Autodesk Fusion 360 part; units mm, degrees
(part 5 of 9)
  line L160 (103.5375, 54.625) -> (115.5375, 54.625)
  arc A163 (116.5375, 53.625) -> (115.5375, 54.625) centre (115.5375, 53.625) ccw
  line L161 (116.5375, 53.625) -> (116.5375, 41.625)
  arc A164 (115.5375, 40.625) -> (116.5375, 41.625) centre (115.5375, 41.625) ccw
  line L162 (115.5375, 40.625) -> (103.5375, 40.625)
  arc A165 (102.5375, 41.625) -> (103.5375, 40.625) centre (103.5375, 41.625) ccw
  line L163 (102.5375, 41.625) -> (102.5375, 53.625)
  arc A166 (251.175, 16.525) -> (250.175, 15.525) centre (251.175, 15.525) ccw
  line L164 (251.175, 16.525) -> (263.175, 16.525)
  arc A167 (264.175, 15.525) -> (263.175, 16.525) centre (263.175, 15.525) ccw
  line L165 (264.175, 15.525) -> (264.175, 3.525)
  arc A168 (263.175, 2.525) -> (264.175, 3.525) centre (263.175, 3.525) ccw
  line L166 (263.175, 2.525) -> (251.175, 2.525)
  arc A169 (250.175, 3.525) -> (251.175, 2.525) centre (251.175, 3.525) ccw
  line L167 (250.175, 3.525) -> (250.175, 15.525)
  arc A170 (123.2563, 72.675) -> (122.2563, 73.675) centre (122.2563, 72.675) ccw
  line L168 (123.2563, 72.675) -> (123.2563, 60.675)
  arc A171 (122.2563, 59.675) -> (123.2563, 60.675) centre (122.2563, 60.675) ccw
  line L169 (122.2563, 59.675) -> (92.0563, 59.675)
  arc A172 (91.0563, 60.675) -> (92.0563, 59.675) centre (92.0563, 60.675) ccw
  line L170 (91.0563, 60.675) -> (91.0563, 72.675)
  arc A173 (92.0563, 73.675) -> (91.0563, 72.675) centre (92.0563, 72.675) ccw
  line L171 (92.0563, 73.675) -> (122.2563, 73.675)
  circle A174 centre (128.588, 37.025) radius 1.25
  circle A175 centre (47.625, 9.525) radius 1.25
  arc A176 (132.1125, 35.575) -> (131.1125, 34.575) centre (132.1125, 34.575) ccw
  line L172 (132.1125, 35.575) -> (144.1125, 35.575)
  arc A177 (145.1125, 34.575) -> (144.1125, 35.575) centre (144.1125, 34.575) ccw
  line L173 (145.1125, 34.575) -> (145.1125, 22.575)
  arc A178 (144.1125, 21.575) -> (145.1125, 22.575) centre (144.1125, 22.575) ccw
  line L174 (144.1125, 21.575) -> (132.1125, 21.575)
  arc A179 (131.1125, 22.575) -> (132.1125, 21.575) centre (132.1125, 22.575) ccw
  line L175 (131.1125, 22.575) -> (131.1125, 34.575)
  arc A180 (94.0125, 35.575) -> (93.0125, 34.575) centre (94.0125, 34.575) ccw
  line L176 (94.0125, 35.575) -> (106.0125, 35.575)
  arc A181 (107.0125, 34.575) -> (106.0125, 35.575) centre (106.0125, 34.575) ccw
  line L177 (107.0125, 34.575) -> (107.0125, 22.575)
  arc A182 (106.0125, 21.575) -> (107.0125, 22.575) centre (106.0125, 22.575) ccw
  line L178 (106.0125, 21.575) -> (94.0125, 21.575)
  arc A183 (93.0125, 22.575) -> (94.0125, 21.575) centre (94.0125, 22.575) ccw
  line L179 (93.0125, 22.575) -> (93.0125, 34.575)
  circle A184 centre (32.525, 66.675) radius 1.25
  line L180 (241.3625, 58.15) -> (241.3625, 73.2)
  arc A185 (241.3625, 73.2) -> (239.8875, 74.675) centre (239.8875, 73.2) ccw
  line L181 (239.8875, 74.675) -> (12.525, 74.675)
  arc A186 (12.525, 74.675) -> (11.05, 73.2) centre (12.525, 73.2) ccw
  line L182 (11.05, 73.2) -> (11.05, 58.15)
  arc A187 (8.525, 55.625) -> (11.05, 58.15) centre (8.525, 58.15) ccw
  line L183 (8.525, 55.625) -> (3, 55.625)
  arc A188 (3, 55.625) -> (1.525, 54.15) centre (3, 54.15) ccw
  line L184 (1.525, 54.15) -> (1.525, 3)
  arc A189 (1.525, 3) -> (3, 1.525) centre (3, 3) ccw
  line L185 (3, 1.525) -> (263.7, 1.525)
  arc A190 (263.7, 1.525) -> (265.175, 3) centre (263.7, 3) ccw
  line L186 (265.175, 3) -> (265.175, 54.15)
  arc A191 (265.175, 54.15) -> (263.7, 55.625) centre (263.7, 54.15) ccw
  line L187 (263.7, 55.625) -> (243.8875, 55.625)
  arc A192 (241.3625, 58.15) -> (243.8875, 55.625) centre (243.8875, 58.15) ccw
  line L188 (163.7375, 72.3724) -> (155.7375, 72.3724)
  line L189 (155.7375, 72.3724) -> (155.7375, 74.675)
  line L190 (156.7375, 75.675) -> (162.7375, 75.675)
  line L191 (163.7375, 74.675) -> (163.7375, 72.3724)
  arc A193 (163.7375, 74.675) -> (162.7375, 75.675) centre (162.7375, 74.675) ccw
  arc A194 (156.7375, 75.675) -> (155.7375, 74.675) centre (156.7375, 74.675) ccw
  line L192 (131.5375, 70.0356) -> (139.5375, 70.0356)
  line L193 (139.5375, 70.0356) -> (139.5375, 74.675)
  line L194 (138.5375, 75.675) -> (132.5375, 75.675)
  line L195 (131.5375, 74.675) -> (131.5375, 70.0356)
  arc A195 (139.5375, 74.675) -> (138.5375, 75.675) centre (138.5375, 74.675) ccw
  arc A196 (132.5375, 75.675) -> (131.5375, 74.675) centre (132.5375, 74.675) ccw
  line L196 (150.1375, 73.675) -> (145.1375, 73.675)
  line L197 (145.1375, 73.675) -> (145.1375, 74.675)
  line L198 (145.1375, 74.675) -> (150.1375, 74.675)
  line L199 (150.1375, 74.675) -> (150.1375, 73.675)
  line L200 (90.0563, 55.625) -> (90.0563, 58.675)
  line L201 (164.7375, 58.675) -> (164.7375, 55.625)
  line L202 (134.1008, 59.675) -> (120, 59.675)
  line L203 (120, 59.675) -> (120, 62.425)
  line L204 (120, 62.425) -> (134.1008, 62.425)
  line L205 (134.1008, 62.425) -> (134.1008, 59.675)
  line L206 (91.0563, 69.6315) -> (99.0563, 69.6315)
  line L207 (99.0563, 69.6315) -> (99.0563, 74.675)
  line L208 (98.0563, 75.675) -> (92.0563, 75.675)
  line L209 (91.0563, 74.675) -> (91.0563, 69.6315)
  line L210 (123.2563, 68.7427) -> (115.2563, 68.7427)
  line L211 (115.2563, 68.7427) -> (115.2563, 74.675)
  line L212 (116.2563, 75.675) -> (122.2563, 75.675)
  line L213 (123.2563, 74.675) -> (123.2563, 68.7427)
  line L214 (109.6563, 73.675) -> (104.6563, 73.675)
  line L215 (104.6563, 73.675) -> (104.6563, 74.675)
  line L216 (104.6563, 74.675) -> (109.6563, 74.675)
  line L217 (109.6563, 74.675) -> (109.6563, 73.675)
  line L218 (91.0563, 61.8134) -> (91.0563, 59.675)
  line L219 (91.0563, 59.675) -> (91.0563, 59.675)
  arc A197 (91.0563, 59.675) -> (90.0563, 58.675) centre (91.0563, 58.675) ccw
  line L220 (92.0563, 59.675) -> (122.2563, 59.675)
  line L221 (163.7375, 61.2223) -> (163.7375, 59.675)
  line L222 (132.5375, 59.675) -> (162.7375, 59.675)
  line L223 (163.7375, 59.675) -> (163.7375, 59.675)
  arc A198 (164.7375, 58.675) -> (163.7375, 59.675) centre (163.7375, 58.675) ccw
  line L224 (159.6875, 52.1672) -> (154.6375, 52.1672)
  line L225 (154.6375, 52.1672) -> (154.6375, 53.625)
  line L226 (155.6375, 54.625) -> (158.6875, 54.625)
  line L227 (159.6875, 53.625) -> (159.6875, 52.1672)
  arc A199 (159.6875, 53.625) -> (158.6875, 54.625) centre (158.6875, 53.625) ccw
  arc A200 (155.6375, 54.625) -> (154.6375, 53.625) centre (155.6375, 53.625) ccw
  line L228 (164.7375, 54.625) -> (160.6875, 54.625)
  line L229 (158.6875, 54.625) -> (155.6375, 54.625)
  line L230 (140.6375, 52.2028) -> (135.5875, 52.2028)
  line L231 (135.5875, 52.2028) -> (135.5875, 53.625)
  line L232 (136.5875, 54.625) -> (139.6375, 54.625)
  line L233 (140.6375, 53.625) -> (140.6375, 52.2028)
  arc A201 (140.6375, 53.625) -> (139.6375, 54.625) centre (139.6375, 53.625) ccw
  arc A202 (136.5875, 54.625) -> (135.5875, 53.625) centre (136.5875, 53.625) ccw
  line L234 (153.6375, 54.625) -> (141.6375, 54.625)
  line L235 (139.6375, 54.625) -> (136.5875, 54.625)
  line L236 (121.5875, 52.4995) -> (116.5375, 52.4995)
  line L237 (116.5375, 52.4995) -> (116.5375, 53.625)
  line L238 (117.5375, 54.625) -> (120.5875, 54.625)
  line L239 (121.5875, 53.625) -> (121.5875, 52.4995)
  arc A203 (121.5875, 53.625) -> (120.5875, 54.625) centre (120.5875, 53.625) ccw
  arc A204 (117.5375, 54.625) -> (116.5375, 53.625) centre (117.5375, 53.625) ccw
  line L240 (134.5875, 54.625) -> (122.5875, 54.625)
  line L241 (120.5875, 54.625) -> (117.5375, 54.625)
  line L242 (102.5375, 52.5305) -> (97.4875, 52.5305)
  line L243 (97.4875, 52.5305) -> (97.4875, 53.625)
  line L244 (98.4875, 54.625) -> (101.5375, 54.625)
  line L245 (102.5375, 53.625) -> (102.5375, 52.5305)
  arc A205 (102.5375, 53.625) -> (101.5375, 54.625) centre (101.5375, 53.625) ccw
  arc A206 (98.4875, 54.625) -> (97.4875, 53.625) centre (98.4875, 53.625) ccw
  line L246 (96.4875, 54.625) -> (90.0563, 54.625)
  line L247 (115.5375, 54.625) -> (103.5375, 54.625)
  line L248 (101.5375, 54.625) -> (98.4875, 54.625)
  arc A207 (123.2563, 74.675) -> (122.2563, 75.675) centre (122.2563, 74.675) ccw
  arc A208 (116.2563, 75.675) -> (115.2563, 74.675) centre (116.2563, 74.675) ccw
  arc A209 (99.0563, 74.675) -> (98.0563, 75.675) centre (98.0563, 74.675) ccw
  arc A210 (92.0563, 75.675) -> (91.0563, 74.675) centre (92.0563, 74.675) ccw
  line L249 (169.1875, 54.625) -> (164.1875, 54.625)
  line L250 (164.7375, 55.625) -> (169.1875, 55.625)
  line L251 (169.1875, 55.625) -> (169.1875, 54.625)
  line L252 (87.9875, 54.625) -> (92.9875, 54.625)
  line L253 (90.0563, 55.625) -> (87.9875, 55.625)
  line L254 (87.9875, 55.625) -> (87.9875, 54.625)
  dimension "d114" = 8
  dimension "d115" = 2
  dimension "d116" = 1
  dimension "d117" = 8
  dimension "d118" = 2
  dimension "d119" = 1
  dimension "d120" = 5
  dimension "d121" = 13.6
  dimension "d122" = 1
  dimension "d123" = 1
  dimension "d124" = 2.75
  dimension "d125" = 8
  dimension "d126" = 2
  dimension "d127" = 8
  dimension "d128" = 2
  dimension "d129" = 5
  dimension "d130" = 13.6
  dimension "d131" = 1
  dimension "d132" = 1
  dimension "d133" = 1
  dimension "d134" = 1
  dimension "d135" = 1
  dimension "d136" = 1
  dimension "d137" = 1
  dimension "d138" = 5
  dimension "d139" = 1
  dimension "d140" = 4.5
  dimension "d141" = 5
  dimension "d142" = 1
  dimension "d143" = 4.5
  constraint horizontal L188
  constraint vertical L189
  constraint horizontal L190
  constraint vertical L191
  constraint coincident L130 L188.start
  constraint tangent L190 A193
  constraint tangent L191 A193
  constraint tangent L189 A194
  constraint tangent L190 A194
  constraint equal A193 A194
  constraint horizontal L192
  constraint vertical L193
  constraint horizontal L194
  constraint vertical L195
  constraint coincident L128 L192.start
  constraint tangent L193 A195
  constraint tangent L194 A195
  constraint tangent L194 A196
  constraint tangent L195 A196
  constraint equal A195 A196
  constraint horizontal L196
  constraint vertical L197
  constraint horizontal L198
  constraint vertical L199
  constraint coincident L129 L196.start
  constraint horizontal L228
  constraint vertical L200
  constraint vertical L201
  constraint coincident L156 L228.start
  constraint horizontal L202
  constraint vertical L203
  constraint horizontal L204
  constraint vertical L205
  constraint coincident L131 L202.start
  constraint horizontal L206
  constraint vertical L207
  constraint horizontal L208
  constraint vertical L209
  constraint coincident L170 L206.start
  constraint horizontal L210
  constraint vertical L211
  constraint horizontal L212
  constraint vertical L213
  constraint coincident L168 L210.start
  constraint horizontal L214
  constraint vertical L215
  constraint horizontal L216
  constraint vertical L217
  constraint coincident L171 L214.start
  constraint coincident L170 L218.start
  constraint parallel L170 L218
  constraint tangent L200 A197
  constraint collinear L220 L222
  constraint coincident L130 L221.start
  constraint parallel L130 L221
  constraint coincident L221.end L222
  constraint tangent L201 A198
  constraint horizontal L224
  constraint vertical L225
  constraint horizontal L226
  constraint vertical L227
  constraint coincident L159 L224.start
  constraint tangent L226 A199
  constraint tangent L227 A199
  constraint tangent L225 A200
  constraint tangent L226 A200
  constraint equal A199 A200
  constraint collinear L228 L229
  constraint collinear L229 L234
  constraint horizontal L230
  constraint vertical L231
  constraint horizontal L232
  constraint vertical L233
  constraint coincident L139 L230.start
  constraint tangent L232 A201
  constraint tangent L233 A201
  constraint tangent L231 A202
  constraint tangent L232 A202
  constraint equal A201 A202
  constraint collinear L234 L235
  constraint collinear L235 L240
  constraint horizontal L236
  constraint vertical L237
  constraint horizontal L238
  constraint vertical L239
  constraint coincident L155 L236.start
  constraint tangent L238 A203
  constraint tangent L239 A203
  constraint tangent L237 A204
  constraint tangent L238 A204
  constraint equal A203 A204
  constraint collinear L240 L241
  constraint collinear L241 L247
  constraint horizontal L242
  constraint vertical L243
  constraint horizontal L244
  constraint vertical L245
  constraint coincident L163 L242.start
  constraint tangent L244 A205
  constraint tangent L245 A205
  constraint tangent L243 A206
  constraint tangent L244 A206
  constraint equal A205 A206
  constraint collinear L246 L247
  constraint collinear L247 L248
  constraint tangent L212 A207
  constraint tangent L213 A207
  constraint tangent L211 A208
  constraint tangent L212 A208
  constraint equal A207 A208
  constraint tangent L207 A209
  constraint tangent L208 A209
  constraint equal A207 A209
  constraint tangent L208 A210
  constraint tangent L209 A210
  constraint equal A207 A210
  constraint horizontal L249
  constraint horizontal L250
  constraint vertical L251
  constraint coincident L156 L249.start
  constraint horizontal L252
  constraint horizontal L253
  constraint vertical L254
  constraint coincident L112 L252.start
  measures "d114" distance of L188.start L188.end
  measures "d115" distance of L129 L190
  measures "d116" radius of A193
  measures "d117" distance of L192.start L192.end
  measures "d118" distance of L129 L194
  measures "d119" radius of A195
  measures "d120" distance of L196.start L196.end
  measures "d121" distance of L130 L199
  measures "d122" distance of L170 L200
  measures "d123" distance of L130 L201
  measures "d124" distance of L202.start L204.end
  measures "d125" distance of L206.start L206.end
  measures "d126" distance of L171 L208
  measures "d127" distance of L210.start L210.end
  measures "d128" distance of L171 L212
  measures "d129" distance of L214.start L214.end
  measures "d130" distance of L168 L217
  measures "d131" radius of A197
  measures "d132" radius of A198
  measures "d133" radius of A199
  measures "d134" radius of A201
  measures "d135" radius of A203
  measures "d136" radius of A205
  measures "d137" radius of A207
  measures "d138" distance of L249.start L249.end
  measures "d139" distance of L249.start L250.end
  measures "d140" distance of L157 L251
  measures "d141" distance of L252.start L252.end
  measures "d142" distance of L252.start L253.end
  measures "d143" distance of L115 L254
extrude "Extrude7" cut sketch "Sketch8" against normal blind 3 contours L112 A113 A133 L131 A138 L136 A139 A154 L152 A155 A158 L156 A162 L160 A163 L169 A172 L200 L201 L202 L218 A197 L220 L221 L222 A198 L226 A199 A200 L228 L229 L232 A201 A202 L234 L235 L238 A203 A204 L240 L241 L244 A205 A206 L246 L247 L248 L249 L250 L251 L252 L253 L254 | A130 L128 L168 A171 L202 L204 | A173 L171 L181 L207 L209 | L171 L181 L214 L215 L216 L217 | A170 L171 L181 L211 L213 | A131 L129 L181 L193 L195 | L129 L181 L196 L197 L198 L199 | L129 A132 L181 L189 L191
sketch "Sketch9" plane through (0, 0, 0) normal (0, -1, 0) x (1, 0, 0)
  arc A0 (241.3625, 73.2) -> (239.8875, 74.675) centre (239.8875, 73.2) ccw
  line L0 (241.3625, 73.2) -> (241.3625, 58.15)
  arc A1 (241.3625, 58.15) -> (243.8875, 55.625) centre (243.8875, 58.15) ccw
  line L1 (243.8875, 55.625) -> (263.7, 55.625)
  arc A2 (265.175, 54.15) -> (263.7, 55.625) centre (263.7, 54.15) ccw
  line L2 (265.175, 54.15) -> (265.175, 3)
  arc A3 (263.7, 1.525) -> (265.175, 3) centre (263.7, 3) ccw
  line L3 (263.7, 1.525) -> (3, 1.525)
  arc A4 (1.525, 3) -> (3, 1.525) centre (3, 3) ccw
  line L4 (1.525, 3) -> (1.525, 54.15)
  arc A5 (3, 55.625) -> (1.525, 54.15) centre (3, 54.15) ccw
  line L5 (3, 55.625) -> (8.525, 55.625)
  arc A6 (8.525, 55.625) -> (11.05, 58.15) centre (8.525, 58.15) ccw
  line L6 (11.05, 58.15) -> (11.05, 73.2)
  arc A7 (12.525, 74.675) -> (11.05, 73.2) centre (12.525, 73.2) ccw
  line L7 (12.525, 74.675) -> (239.8875, 74.675)
  arc A8 (266.7, 54.15) -> (263.7, 57.15) centre (263.7, 54.15) ccw
  line L8 (263.7, 57.15) -> (243.8875, 57.15)
  arc A9 (242.8875, 58.15) -> (243.8875, 57.15) centre (243.8875, 58.15) ccw
  line L9 (242.8875, 58.15) -> (242.8875, 73.2)
  arc A10 (242.8875, 73.2) -> (239.8875, 76.2) centre (239.8875, 73.2) ccw
  line L10 (239.8875, 76.2) -> (12.525, 76.2)
  arc A11 (12.525, 76.2) -> (9.525, 73.2) centre (12.525, 73.2) ccw
  line L11 (9.525, 73.2) -> (9.525, 58.15)
  arc A12 (8.525, 57.15) -> (9.525, 58.15) centre (8.525, 58.15) ccw
  line L12 (8.525, 57.15) -> (3, 57.15)
  arc A13 (3, 57.15) -> (0, 54.15) centre (3, 54.15) ccw
  line L13 (0, 54.15) -> (0, 3)
  arc A14 (0, 3) -> (3, 0) centre (3, 3) ccw
  line L14 (3, 0) -> (263.7, 0)
  arc A15 (263.7, 0) -> (266.7, 3) centre (263.7, 3) ccw
  line L15 (266.7, 3) -> (266.7, 54.15)
  line L16 (163.7375, 71.7638) -> (155.7375, 71.7638)
  line L17 (155.7375, 71.7638) -> (155.7375, 75.675)
  line L18 (155.7375, 75.675) -> (163.7375, 75.675)
  line L19 (163.7375, 75.675) -> (163.7375, 71.7638)
  line L20 (163.7375, 60.675) -> (163.7375, 72.675)
  line L21 (162.7375, 73.675) -> (155.7375, 73.675)
  line L22 (131.5375, 70.9794) -> (139.5375, 70.9794)
  line L23 (139.5375, 70.9794) -> (139.5375, 75.675)
  line L24 (139.5375, 75.675) -> (131.5375, 75.675)
  line L25 (131.5375, 75.675) -> (131.5375, 70.9794)
  line L26 (131.5375, 72.675) -> (131.5375, 60.675)
  line L27 (139.5375, 73.675) -> (132.5375, 73.675)
  line L28 (123.2563, 71.4279) -> (115.2563, 71.4279)
  line L29 (115.2563, 71.4279) -> (115.2563, 75.675)
  line L30 (115.2563, 75.675) -> (123.2563, 75.675)
  line L31 (123.2563, 75.675) -> (123.2563, 71.4279)
  line L32 (123.2563, 60.675) -> (123.2563, 72.675)
  line L33 (122.2563, 73.675) -> (115.2563, 73.675)
  line L34 (91.0563, 72.2259) -> (99.0563, 72.2259)
  line L35 (99.0563, 72.2259) -> (99.0563, 75.675)
  line L36 (99.0563, 75.675) -> (91.0563, 75.675)
  line L37 (91.0563, 75.675) -> (91.0563, 72.2259)
  line L38 (91.0563, 59.675) -> (91.0563, 74.675)
  line L39 (99.0563, 73.675) -> (92.0563, 73.675)
  dimension "d146" = 8
  dimension "d147" = 2
  dimension "d148" = 8
  dimension "d149" = 2
  dimension "d150" = 8
  dimension "d151" = 2
  dimension "d152" = 8
  dimension "d153" = 2
  constraint horizontal L16
  constraint vertical L17
  constraint horizontal L18
  constraint vertical L19
  constraint coincident L16.start L20
  constraint horizontal L22
  constraint vertical L23
  constraint horizontal L24
  constraint vertical L25
  constraint coincident L22.start L26
  constraint horizontal L28
  constraint vertical L29
  constraint horizontal L30
  constraint vertical L31
  constraint coincident L28.start L32
  constraint horizontal L34
  constraint vertical L35
  constraint horizontal L36
  constraint vertical L37
  constraint coincident L34.start L38
  measures "d146" distance of L16.start L16.end
  measures "d147" distance of L18 L21
  measures "d148" distance of L22.start L22.end
  measures "d149" distance of L24 L27
  measures "d150" distance of L28.start L28.end
  measures "d151" distance of L30 L33
  measures "d152" distance of L34.start L34.end
  measures "d153" distance of L36 L39
extrude "Extrude8" cut sketch "Sketch9" against normal blind 3.6 contours L7 L17 L18 L19 | L7 L23 L24 L25 | L7 L29 L30 L31 | L7 L35 L36 L37
fillet "Fillet3" radius 1 12 edges at (163.7375, 1.8, 75.675) (155.7375, 1.8, 75.675) (150.1375, 2.1, 74.675) (145.1375, 2.1, 74.675) (139.5375, 1.8, 75.675) (131.5375, 1.8, 75.675) (123.2563, 1.8, 75.675) (115.2563, 1.8, 75.675) (109.6563, 2.1, 74.675) (104.6563, 2.1, 74.675) (99.0563, 1.8, 75.675) (91.0563, 1.8, 75.675)
fillet "Fillet4" radius 1 1 edges at (87.9875, 2.1, 55.625)
fillet "Fillet5" radius 1 1 edges at (169.1875, 2.1, 55.625)
sketch "Sketch10" plane through (0, 0.6, 0) normal (0, -1, 0) x (1, 0, 0)
  circle A0 centre (32.525, 66.675) radius 1.25
  arc A1 (94.0125, 35.575) -> (93.0125, 34.575) centre (94.0125, 34.575) ccw
  line L0 (94.0125, 35.575) -> (106.0125, 35.575)
  arc A2 (107.0125, 34.575) -> (106.0125, 35.575) centre (106.0125, 34.575) ccw
  line L1 (107.0125, 34.575) -> (107.0125, 22.575)
  arc A3 (106.0125, 21.575) -> (107.0125, 22.575) centre (106.0125, 22.575) ccw
  line L2 (106.0125, 21.575) -> (94.0125, 21.575)
  arc A4 (93.0125, 22.575) -> (94.0125, 21.575) centre (94.0125, 22.575) ccw
  line L3 (93.0125, 22.575) -> (93.0125, 34.575)
  arc A5 (132.1125, 35.575) -> (131.1125, 34.575) centre (132.1125, 34.575) ccw
  line L4 (132.1125, 35.575) -> (144.1125, 35.575)
  arc A6 (145.1125, 34.575) -> (144.1125, 35.575) centre (144.1125, 34.575) ccw
  line L5 (145.1125, 34.575) -> (145.1125, 22.575)
  arc A7 (144.1125, 21.575) -> (145.1125, 22.575) centre (144.1125, 22.575) ccw
  line L6 (144.1125, 21.575) -> (132.1125, 21.575)
  arc A8 (131.1125, 22.575) -> (132.1125, 21.575) centre (132.1125, 22.575) ccw
  line L7 (131.1125, 22.575) -> (131.1125, 34.575)
  circle A9 centre (47.625, 9.525) radius 1.25
  circle A10 centre (128.588, 37.025) radius 1.25
  arc A11 (251.175, 16.525) -> (250.175, 15.525) centre (251.175, 15.525) ccw
  line L8 (251.175, 16.525) -> (263.175, 16.525)
  arc A12 (264.175, 15.525) -> (263.175, 16.525) centre (263.175, 15.525) ccw
  line L9 (264.175, 15.525) -> (264.175, 3.525)
  arc A13 (263.175, 2.525) -> (264.175, 3.525) centre (263.175, 3.525) ccw
  line L10 (263.175, 2.525) -> (251.175, 2.525)
  arc A14 (250.175, 3.525) -> (251.175, 2.525) centre (251.175, 3.525) ccw
  line L11 (250.175, 3.525) -> (250.175, 15.525)
  arc A15 (217.8375, 54.625) -> (216.8375, 53.625) centre (217.8375, 53.625) ccw
  line L12 (217.8375, 54.625) -> (229.8375, 54.625)
  arc A16 (230.8375, 53.625) -> (229.8375, 54.625) centre (229.8375, 53.625) ccw
  line L13 (230.8375, 53.625) -> (230.8375, 41.625)
  arc A17 (229.8375, 40.625) -> (230.8375, 41.625) centre (229.8375, 41.625) ccw
  line L14 (229.8375, 40.625) -> (217.8375, 40.625)
  arc A18 (216.8375, 41.625) -> (217.8375, 40.625) centre (217.8375, 41.625) ccw
  line L15 (216.8375, 41.625) -> (216.8375, 53.625)
  arc A19 (179.7375, 54.625) -> (178.7375, 53.625) centre (179.7375, 53.625) ccw
  line L16 (179.7375, 54.625) -> (191.7375, 54.625)
  arc A20 (192.7375, 53.625) -> (191.7375, 54.625) centre (191.7375, 53.625) ccw
  line L17 (192.7375, 53.625) -> (192.7375, 41.625)
  arc A21 (191.7375, 40.625) -> (192.7375, 41.625) centre (191.7375, 41.625) ccw
  line L18 (191.7375, 40.625) -> (179.7375, 40.625)
  arc A22 (178.7375, 41.625) -> (179.7375, 40.625) centre (179.7375, 41.625) ccw
  line L19 (178.7375, 41.625) -> (178.7375, 53.625)
  arc A23 (108.3, 16.525) -> (107.3, 15.525) centre (108.3, 15.525) ccw
  line L20 (108.3, 16.525) -> (120.3, 16.525)
  arc A24 (121.3, 15.525) -> (120.3, 16.525) centre (120.3, 15.525) ccw
  line L21 (121.3, 15.525) -> (121.3, 3.525)
  arc A25 (120.3, 2.525) -> (121.3, 3.525) centre (120.3, 3.525) ccw
  line L22 (120.3, 2.525) -> (108.3, 2.525)
  arc A26 (107.3, 3.525) -> (108.3, 2.525) centre (108.3, 3.525) ccw
  line L23 (107.3, 3.525) -> (107.3, 15.525)
  arc A27 (5.3312, 41.625) -> (6.3312, 40.625) centre (6.3312, 41.625) ccw
  line L24 (5.3312, 41.625) -> (5.3313, 53.625)
  arc A28 (6.3312, 54.625) -> (5.3312, 53.625) centre (6.3312, 53.625) ccw
  line L25 (6.3312, 54.625) -> (36.5313, 54.625)
  arc A29 (37.5312, 53.625) -> (36.5313, 54.625) centre (36.5313, 53.625) ccw
  line L26 (37.5312, 53.625) -> (37.5313, 41.625)
  arc A30 (36.5313, 40.625) -> (37.5312, 41.625) centre (36.5313, 41.625) ccw
  line L27 (36.5313, 40.625) -> (6.3312, 40.625)
  arc A31 (203.55, 16.525) -> (202.55, 15.525) centre (203.55, 15.525) ccw
  line L28 (203.55, 16.525) -> (215.55, 16.525)
  arc A32 (216.55, 15.525) -> (215.55, 16.525) centre (215.55, 15.525) ccw
  line L29 (216.55, 15.525) -> (216.55, 3.525)
  arc A33 (215.55, 2.525) -> (216.55, 3.525) centre (215.55, 3.525) ccw
  line L30 (215.55, 2.525) -> (203.55, 2.525)
  arc A34 (202.55, 3.525) -> (203.55, 2.525) centre (203.55, 3.525) ccw
  line L31 (202.55, 3.525) -> (202.55, 15.525)
  circle A35 centre (245.269, 9.525) radius 1.25
  circle A36 centre (220.025, 66.675) radius 1.25
  arc A37 (189.2625, 35.575) -> (188.2625, 34.575) centre (189.2625, 34.575) ccw
  line L32 (189.2625, 35.575) -> (201.2625, 35.575)
  arc A38 (202.2625, 34.575) -> (201.2625, 35.575) centre (201.2625, 34.575) ccw
  line L33 (202.2625, 34.575) -> (202.2625, 22.575)
  arc A39 (201.2625, 21.575) -> (202.2625, 22.575) centre (201.2625, 22.575) ccw
  line L34 (201.2625, 21.575) -> (189.2625, 21.575)
  arc A40 (188.2625, 22.575) -> (189.2625, 21.575) centre (189.2625, 22.575) ccw
  line L35 (188.2625, 22.575) -> (188.2625, 34.575)
  arc A41 (146.4, 16.525) -> (145.4, 15.525) centre (146.4, 15.525) ccw
  line L36 (146.4, 16.525) -> (158.4, 16.525)
  arc A42 (159.4, 15.525) -> (158.4, 16.525) centre (158.4, 15.525) ccw
  line L37 (159.4, 15.525) -> (159.4, 3.525)
  arc A43 (158.4, 2.525) -> (159.4, 3.525) centre (158.4, 3.525) ccw
  line L38 (158.4, 2.525) -> (146.4, 2.525)
  arc A44 (145.4, 3.525) -> (146.4, 2.525) centre (146.4, 3.525) ccw
  line L39 (145.4, 3.525) -> (145.4, 15.525)
  arc A45 (113.0625, 35.575) -> (112.0625, 34.575) centre (113.0625, 34.575) ccw
  line L40 (113.0625, 35.575) -> (125.0625, 35.575)
  arc A46 (126.0625, 34.575) -> (125.0625, 35.575) centre (125.0625, 34.575) ccw
  line L41 (126.0625, 34.575) -> (126.0625, 22.575)
  arc A47 (125.0625, 21.575) -> (126.0625, 22.575) centre (125.0625, 22.575) ccw
  line L42 (125.0625, 21.575) -> (113.0625, 21.575)
  arc A48 (112.0625, 22.575) -> (113.0625, 21.575) centre (113.0625, 22.575) ccw
  line L43 (112.0625, 22.575) -> (112.0625, 34.575)
  arc A49 (127.35, 16.525) -> (126.35, 15.525) centre (127.35, 15.525) ccw
  line L44 (127.35, 16.525) -> (139.35, 16.525)
  arc A50 (140.35, 15.525) -> (139.35, 16.525) centre (139.35, 15.525) ccw
  line L45 (140.35, 15.525) -> (140.35, 3.525)
  arc A51 (139.35, 2.525) -> (140.35, 3.525) centre (139.35, 3.525) ccw
  line L46 (139.35, 2.525) -> (127.35, 2.525)
  arc A52 (126.35, 3.525) -> (127.35, 2.525) centre (127.35, 3.525) ccw
  line L47 (126.35, 3.525) -> (126.35, 15.525)
  arc A53 (170.2125, 35.575) -> (169.2125, 34.575) centre (170.2125, 34.575) ccw
  line L48 (170.2125, 35.575) -> (182.2125, 35.575)
  arc A54 (183.2125, 34.575) -> (182.2125, 35.575) centre (182.2125, 34.575) ccw
  line L49 (183.2125, 34.575) -> (183.2125, 22.575)
  arc A55 (182.2125, 21.575) -> (183.2125, 22.575) centre (182.2125, 22.575) ccw
  line L50 (182.2125, 21.575) -> (170.2125, 21.575)
  arc A56 (169.2125, 22.575) -> (170.2125, 21.575) centre (170.2125, 22.575) ccw
  line L51 (169.2125, 22.575) -> (169.2125, 34.575)
  arc A57 (224.9813, 73.675) -> (223.9813, 72.675) centre (224.9813, 72.675) ccw
  line L52 (224.9813, 73.675) -> (236.9813, 73.675)
  arc A58 (237.9812, 72.675) -> (236.9813, 73.675) centre (236.9813, 72.675) ccw
  line L53 (237.9812, 72.675) -> (237.9813, 60.675)
  arc A59 (236.9813, 59.675) -> (237.9813, 60.675) centre (236.9813, 60.675) ccw
  line L54 (236.9813, 59.675) -> (224.9813, 59.675)
  arc A60 (223.9812, 60.675) -> (224.9813, 59.675) centre (224.9813, 60.675) ccw
  line L55 (223.9812, 60.675) -> (223.9813, 72.675)
  arc A61 (198.7875, 54.625) -> (197.7875, 53.625) centre (198.7875, 53.625) ccw
  line L56 (198.7875, 54.625) -> (210.7875, 54.625)
  arc A62 (211.7875, 53.625) -> (210.7875, 54.625) centre (210.7875, 53.625) ccw
  line L57 (211.7875, 53.625) -> (211.7875, 41.625)
  arc A63 (210.7875, 40.625) -> (211.7875, 41.625) centre (210.7875, 41.625) ccw
  line L58 (210.7875, 40.625) -> (198.7875, 40.625)
  arc A64 (197.7875, 41.625) -> (198.7875, 40.625) centre (198.7875, 41.625) ccw
  line L59 (197.7875, 41.625) -> (197.7875, 53.625)
  arc A65 (51.15, 16.525) -> (50.15, 15.525) centre (51.15, 15.525) ccw
  line L60 (51.15, 16.525) -> (63.15, 16.525)
  arc A66 (64.15, 15.525) -> (63.15, 16.525) centre (63.15, 15.525) ccw
  line L61 (64.15, 15.525) -> (64.15, 3.525)
  arc A67 (63.15, 2.525) -> (64.15, 3.525) centre (63.15, 3.525) ccw
  line L62 (63.15, 2.525) -> (51.15, 2.525)
  arc A68 (50.15, 3.525) -> (51.15, 2.525) centre (51.15, 3.525) ccw
  line L63 (50.15, 3.525) -> (50.15, 15.525)
  arc A69 (8.2875, 16.525) -> (7.2875, 15.525) centre (8.2875, 15.525) ccw
  line L64 (8.2875, 16.525) -> (20.2875, 16.525)
  arc A70 (21.2875, 15.525) -> (20.2875, 16.525) centre (20.2875, 15.525) ccw
  line L65 (21.2875, 15.525) -> (21.2875, 3.525)
  arc A71 (20.2875, 2.525) -> (21.2875, 3.525) centre (20.2875, 3.525) ccw
  line L66 (20.2875, 2.525) -> (8.2875, 2.525)
  arc A72 (7.2875, 3.525) -> (8.2875, 2.525) centre (8.2875, 3.525) ccw
  line L67 (7.2875, 3.525) -> (7.2875, 15.525)
  arc A73 (208.3125, 35.575) -> (207.3125, 34.575) centre (208.3125, 34.575) ccw
  line L68 (208.3125, 35.575) -> (220.3125, 35.575)
  arc A74 (221.3125, 34.575) -> (220.3125, 35.575) centre (220.3125, 34.575) ccw
  line L69 (221.3125, 34.575) -> (221.3125, 22.575)
  arc A75 (220.3125, 21.575) -> (221.3125, 22.575) centre (220.3125, 22.575) ccw
  line L70 (220.3125, 21.575) -> (208.3125, 21.575)
  arc A76 (207.3125, 22.575) -> (208.3125, 21.575) centre (208.3125, 22.575) ccw
  line L71 (207.3125, 22.575) -> (207.3125, 34.575)
  arc A77 (227.3625, 16.525) -> (226.3625, 15.525) centre (227.3625, 15.525) ccw
  line L72 (227.3625, 16.525) -> (239.3625, 16.525)
  arc A78 (240.3625, 15.525) -> (239.3625, 16.525) centre (239.3625, 15.525) ccw
  line L73 (240.3625, 15.525) -> (240.3625, 3.525)
  arc A79 (239.3625, 2.525) -> (240.3625, 3.525) centre (239.3625, 3.525) ccw
  line L74 (239.3625, 2.525) -> (227.3625, 2.525)
  arc A80 (226.3625, 3.525) -> (227.3625, 2.525) centre (227.3625, 3.525) ccw
  line L75 (226.3625, 3.525) -> (226.3625, 15.525)
  arc A81 (36.8625, 35.575) -> (35.8625, 34.575) centre (36.8625, 34.575) ccw
  line L76 (36.8625, 35.575) -> (48.8625, 35.575)
  arc A82 (49.8625, 34.575) -> (48.8625, 35.575) centre (48.8625, 34.575) ccw
  line L77 (49.8625, 34.575) -> (49.8625, 22.575)
  arc A83 (48.8625, 21.575) -> (49.8625, 22.575) centre (48.8625, 22.575) ccw
  line L78 (48.8625, 21.575) -> (36.8625, 21.575)
  arc A84 (35.8625, 22.575) -> (36.8625, 21.575) centre (36.8625, 22.575) ccw
  line L79 (35.8625, 22.575) -> (35.8625, 34.575)
  arc A85 (74.9625, 35.575) -> (73.9625, 34.575) centre (74.9625, 34.575) ccw
  line L80 (74.9625, 35.575) -> (86.9625, 35.575)
  arc A86 (87.9625, 34.575) -> (86.9625, 35.575) centre (86.9625, 34.575) ccw
  line L81 (87.9625, 34.575) -> (87.9625, 22.575)
  arc A87 (86.9625, 21.575) -> (87.9625, 22.575) centre (86.9625, 22.575) ccw
  line L82 (86.9625, 21.575) -> (74.9625, 21.575)
  arc A88 (73.9625, 22.575) -> (74.9625, 21.575) centre (74.9625, 22.575) ccw
  line L83 (73.9625, 22.575) -> (73.9625, 34.575)
  arc A89 (41.625, 73.675) -> (40.625, 72.675) centre (41.625, 72.675) ccw
  line L84 (41.625, 73.675) -> (53.625, 73.675)
  arc A90 (54.625, 72.675) -> (53.625, 73.675) centre (53.625, 72.675) ccw
  line L85 (54.625, 72.675) -> (54.625, 60.675)
  arc A91 (53.625, 59.675) -> (54.625, 60.675) centre (53.625, 60.675) ccw
  line L86 (53.625, 59.675) -> (41.625, 59.675)
  arc A92 (40.625, 60.675) -> (41.625, 59.675) centre (41.625, 60.675) ccw
  line L87 (40.625, 60.675) -> (40.625, 72.675)
  arc A93 (89.25, 16.525) -> (88.25, 15.525) centre (89.25, 15.525) ccw
  line L88 (89.25, 16.525) -> (101.25, 16.525)
  arc A94 (102.25, 15.525) -> (101.25, 16.525) centre (101.25, 15.525) ccw
  line L89 (102.25, 15.525) -> (102.25, 3.525)
  arc A95 (101.25, 2.525) -> (102.25, 3.525) centre (101.25, 3.525) ccw
  line L90 (101.25, 2.525) -> (89.25, 2.525)
  arc A96 (88.25, 3.525) -> (89.25, 2.525) centre (89.25, 3.525) ccw
  line L91 (88.25, 3.525) -> (88.25, 15.525)
  arc A97 (151.1625, 35.575) -> (150.1625, 34.575) centre (151.1625, 34.575) ccw
  line L92 (151.1625, 35.575) -> (163.1625, 35.575)
  arc A98 (164.1625, 34.575) -> (163.1625, 35.575) centre (163.1625, 34.575) ccw
  line L93 (164.1625, 34.575) -> (164.1625, 22.575)
  arc A99 (163.1625, 21.575) -> (164.1625, 22.575) centre (163.1625, 22.575) ccw
  line L94 (163.1625, 21.575) -> (151.1625, 21.575)
  arc A100 (150.1625, 22.575) -> (151.1625, 21.575) centre (151.1625, 22.575) ccw
  line L95 (150.1625, 22.575) -> (150.1625, 34.575)
  arc A101 (172.5938, 73.675) -> (171.5938, 72.675) centre (172.5938, 72.675) ccw
  line L96 (172.5938, 73.675) -> (184.5938, 73.675)
  arc A102 (185.5937, 72.675) -> (184.5938, 73.675) centre (184.5937, 72.675) ccw
  line L97 (185.5937, 72.675) -> (185.5937, 60.675)
  arc A103 (184.5938, 59.675) -> (185.5937, 60.675) centre (184.5938, 60.675) ccw
  line L98 (184.5938, 59.675) -> (172.5937, 59.675)
  arc A104 (171.5938, 60.675) -> (172.5938, 59.675) centre (172.5938, 60.675) ccw
  line L99 (171.5937, 60.675) -> (171.5938, 72.675)
  arc A105 (10.6688, 35.575) -> (9.6688, 34.575) centre (10.6688, 34.575) ccw
  line L100 (10.6688, 35.575) -> (22.6687, 35.575)
  arc A106 (23.6687, 34.575) -> (22.6687, 35.575) centre (22.6687, 34.575) ccw
  line L101 (23.6687, 34.575) -> (23.6688, 22.575)
  arc A107 (22.6687, 21.575) -> (23.6688, 22.575) centre (22.6688, 22.575) ccw
  line L102 (22.6687, 21.575) -> (10.6688, 21.575)
  arc A108 (9.6687, 22.575) -> (10.6688, 21.575) centre (10.6687, 22.575) ccw
  line L103 (9.6687, 22.575) -> (9.6688, 34.575)
  arc A109 (70.2, 16.525) -> (69.2, 15.525) centre (70.2, 15.525) ccw
  line L104 (70.2, 16.525) -> (82.2, 16.525)
  arc A110 (83.2, 15.525) -> (82.2, 16.525) centre (82.2, 15.525) ccw
  line L105 (83.2, 15.525) -> (83.2, 3.525)
  arc A111 (82.2, 2.525) -> (83.2, 3.525) centre (82.2, 3.525) ccw
  line L106 (82.2, 2.525) -> (70.2, 2.525)
  arc A112 (69.2, 3.525) -> (70.2, 2.525) centre (70.2, 3.525) ccw
  line L107 (69.2, 3.525) -> (69.2, 15.525)
  arc A113 (46.3875, 54.625) -> (45.3875, 53.625) centre (46.3875, 53.625) ccw
  line L108 (46.3875, 54.625) -> (58.3875, 54.625)
  arc A114 (59.3875, 53.625) -> (58.3875, 54.625) centre (58.3875, 53.625) ccw
  line L109 (59.3875, 53.625) -> (59.3875, 41.625)
  arc A115 (58.3875, 40.625) -> (59.3875, 41.625) centre (58.3875, 41.625) ccw
  line L110 (58.3875, 40.625) -> (46.3875, 40.625)
  arc A116 (45.3875, 41.625) -> (46.3875, 40.625) centre (46.3875, 41.625) ccw
  line L111 (45.3875, 41.625) -> (45.3875, 53.625)
  arc A117 (55.9125, 35.575) -> (54.9125, 34.575) centre (55.9125, 34.575) ccw
  line L112 (55.9125, 35.575) -> (67.9125, 35.575)
  arc A118 (68.9125, 34.575) -> (67.9125, 35.575) centre (67.9125, 34.575) ccw
  line L113 (68.9125, 34.575) -> (68.9125, 22.575)
  arc A119 (67.9125, 21.575) -> (68.9125, 22.575) centre (67.9125, 22.575) ccw
  line L114 (67.9125, 21.575) -> (55.9125, 21.575)
  arc A120 (54.9125, 22.575) -> (55.9125, 21.575) centre (55.9125, 22.575) ccw
  line L115 (54.9125, 22.575) -> (54.9125, 34.575)
  arc A121 (45.1, 15.525) -> (44.1, 16.525) centre (44.1, 15.525) ccw
  line L116 (45.1, 15.525) -> (45.1, 3.525)
  arc A122 (44.1, 2.525) -> (45.1, 3.525) centre (44.1, 3.525) ccw
  line L117 (44.1, 2.525) -> (32.1, 2.525)
  arc A123 (31.1, 3.525) -> (32.1, 2.525) centre (32.1, 3.525) ccw
  line L118 (31.1, 3.525) -> (31.1, 15.525)
  arc A124 (32.1, 16.525) -> (31.1, 15.525) centre (32.1, 15.525) ccw
  line L119 (32.1, 16.525) -> (44.1, 16.525)
  arc A125 (184.5, 16.525) -> (183.5, 15.525) centre (184.5, 15.525) ccw
  line L120 (184.5, 16.525) -> (196.5, 16.525)
  arc A126 (197.5, 15.525) -> (196.5, 16.525) centre (196.5, 15.525) ccw
  line L121 (197.5, 15.525) -> (197.5, 3.525)
  arc A127 (196.5, 2.525) -> (197.5, 3.525) centre (196.5, 3.525) ccw
  line L122 (196.5, 2.525) -> (184.5, 2.525)
  arc A128 (183.5, 3.525) -> (184.5, 2.525) centre (184.5, 3.525) ccw
  line L123 (183.5, 3.525) -> (183.5, 15.525)
  arc A129 (261.3688, 34.575) -> (260.3688, 35.575) centre (260.3688, 34.575) ccw
  line L124 (261.3688, 34.575) -> (261.3688, 22.575)
  arc A130 (260.3688, 21.575) -> (261.3688, 22.575) centre (260.3688, 22.575) ccw
  line L125 (260.3688, 21.575) -> (230.1688, 21.575)
  arc A131 (229.1688, 22.575) -> (230.1688, 21.575) centre (230.1688, 22.575) ccw
  line L126 (229.1688, 22.575) -> (229.1688, 34.575)
  arc A132 (230.1688, 35.575) -> (229.1688, 34.575) centre (230.1688, 34.575) ccw
  line L127 (230.1688, 35.575) -> (260.3688, 35.575)
  arc A133 (67.8188, 73.675) -> (66.8188, 72.675) centre (67.8188, 72.675) ccw
  line L128 (67.8188, 73.675) -> (79.8188, 73.675)
  arc A134 (80.8188, 72.675) -> (79.8188, 73.675) centre (79.8188, 72.675) ccw
  line L129 (80.8187, 72.675) -> (80.8187, 60.675)
  arc A135 (79.8188, 59.675) -> (80.8188, 60.675) centre (79.8188, 60.675) ccw
  line L130 (79.8188, 59.675) -> (67.8188, 59.675)
  arc A136 (66.8188, 60.675) -> (67.8188, 59.675) centre (67.8188, 60.675) ccw
  line L131 (66.8188, 60.675) -> (66.8188, 72.675)
  arc A137 (165.45, 16.525) -> (164.45, 15.525) centre (165.45, 15.525) ccw
  line L132 (165.45, 16.525) -> (177.45, 16.525)
  arc A138 (178.45, 15.525) -> (177.45, 16.525) centre (177.45, 15.525) ccw
  line L133 (178.45, 15.525) -> (178.45, 3.525)
  arc A139 (177.45, 2.525) -> (178.45, 3.525) centre (177.45, 3.525) ccw
  line L134 (177.45, 2.525) -> (165.45, 2.525)
  arc A140 (164.45, 3.525) -> (165.45, 2.525) centre (165.45, 3.525) ccw
  line L135 (164.45, 3.525) -> (164.45, 15.525)
  arc A141 (14.4313, 60.675) -> (15.4313, 59.675) centre (15.4313, 60.675) ccw
  line L136 (14.4313, 60.675) -> (14.4313, 72.675)
  arc A142 (15.4313, 73.675) -> (14.4313, 72.675) centre (15.4313, 72.675) ccw
  line L137 (15.4313, 73.675) -> (27.4313, 73.675)
  arc A143 (28.4312, 72.675) -> (27.4313, 73.675) centre (27.4312, 72.675) ccw
  line L138 (28.4312, 72.675) -> (28.4313, 60.675)
  arc A144 (27.4313, 59.675) -> (28.4313, 60.675) centre (27.4313, 60.675) ccw
  line L139 (27.4313, 59.675) -> (15.4313, 59.675)
  arc A145 (244.0312, 54.625) -> (243.0313, 53.625) centre (244.0312, 53.625) ccw
  line L140 (244.0312, 54.625) -> (256.0312, 54.625)
  arc A146 (257.0312, 53.625) -> (256.0312, 54.625) centre (256.0312, 53.625) ccw
  line L141 (257.0312, 53.625) -> (257.0312, 41.625)
  arc A147 (256.0312, 40.625) -> (257.0312, 41.625) centre (256.0312, 41.625) ccw
  line L142 (256.0312, 40.625) -> (244.0312, 40.625)
  arc A148 (243.0313, 41.625) -> (244.0312, 40.625) centre (244.0312, 41.625) ccw
  line L143 (243.0312, 41.625) -> (243.0312, 53.625)
  arc A149 (198.7875, 73.675) -> (197.7875, 72.675) centre (198.7875, 72.675) ccw
  line L144 (198.7875, 73.675) -> (210.7875, 73.675)
  arc A150 (211.7875, 72.675) -> (210.7875, 73.675) centre (210.7875, 72.675) ccw
  line L145 (211.7875, 72.675) -> (211.7875, 60.675)
  arc A151 (210.7875, 59.675) -> (211.7875, 60.675) centre (210.7875, 60.675) ccw
  line L146 (210.7875, 59.675) -> (198.7875, 59.675)
  arc A152 (197.7875, 60.675) -> (198.7875, 59.675) centre (198.7875, 60.675) ccw
  line L147 (197.7875, 60.675) -> (197.7875, 72.675)
  arc A153 (65.4375, 54.625) -> (64.4375, 53.625) centre (65.4375, 53.625) ccw
  line L148 (65.4375, 54.625) -> (77.4375, 54.625)
  arc A154 (78.4375, 53.625) -> (77.4375, 54.625) centre (77.4375, 53.625) ccw
  line L149 (78.4375, 53.625) -> (78.4375, 41.625)
  arc A155 (77.4375, 40.625) -> (78.4375, 41.625) centre (77.4375, 41.625) ccw
  line L150 (77.4375, 40.625) -> (65.4375, 40.625)
  arc A156 (64.4375, 41.625) -> (65.4375, 40.625) centre (65.4375, 41.625) ccw
  line L151 (64.4375, 41.625) -> (64.4375, 53.625)
  arc A157 (155.6375, 54.625) -> (154.6375, 53.625) centre (155.6375, 53.625) ccw
  line L152 (154.6375, 53.625) -> (154.6375, 41.625)
  arc A158 (153.6375, 40.625) -> (154.6375, 41.625) centre (153.6375, 41.625) ccw
  line L153 (153.6375, 40.625) -> (141.6375, 40.625)
  arc A159 (140.6375, 41.625) -> (141.6375, 40.625) centre (141.6375, 41.625) ccw
  line L154 (140.6375, 41.625) -> (140.6375, 53.625)
  arc A160 (140.6375, 53.625) -> (139.6375, 54.625) centre (139.6375, 53.625) ccw
  line L155 (139.6375, 54.625) -> (136.5875, 54.625)
  arc A161 (136.5875, 54.625) -> (135.5875, 53.625) centre (136.5875, 53.625) ccw
  line L156 (135.5875, 53.625) -> (135.5875, 41.625)
  arc A162 (134.5875, 40.625) -> (135.5875, 41.625) centre (134.5875, 41.625) ccw
  line L157 (134.5875, 40.625) -> (122.5875, 40.625)
  arc A163 (121.5875, 41.625) -> (122.5875, 40.625) centre (122.5875, 41.625) ccw
  line L158 (121.5875, 41.625) -> (121.5875, 53.625)
  arc A164 (121.5875, 53.625) -> (120.5875, 54.625) centre (120.5875, 53.625) ccw
  line L159 (120.5875, 54.625) -> (117.5375, 54.625)
  arc A165 (117.5375, 54.625) -> (116.5375, 53.625) centre (117.5375, 53.625) ccw
  line L160 (116.5375, 53.625) -> (116.5375, 41.625)
  arc A166 (115.5375, 40.625) -> (116.5375, 41.625) centre (115.5375, 41.625) ccw
  line L161 (115.5375, 40.625) -> (103.5375, 40.625)
  arc A167 (102.5375, 41.625) -> (103.5375, 40.625) centre (103.5375, 41.625) ccw
  line L162 (102.5375, 41.625) -> (102.5375, 53.625)
  arc A168 (102.5375, 53.625) -> (101.5375, 54.625) centre (101.5375, 53.625) ccw
  line L163 (101.5375, 54.625) -> (98.4875, 54.625)
  arc A169 (98.4875, 54.625) -> (97.4875, 53.625) centre (98.4875, 53.625) ccw
  line L164 (97.4875, 53.625) -> (97.4875, 41.625)
  arc A170 (96.4875, 40.625) -> (97.4875, 41.625) centre (96.4875, 41.625) ccw
  line L165 (96.4875, 40.625) -> (84.4875, 40.625)
  arc A171 (83.4875, 41.625) -> (84.4875, 40.625) centre (84.4875, 41.625) ccw
  line L166 (83.4875, 41.625) -> (83.4875, 53.625)
  arc A172 (84.4875, 54.625) -> (83.4875, 53.625) centre (84.4875, 53.625) ccw
  line L167 (84.4875, 54.625) -> (87.9875, 54.625)
  arc A173 (88.9875, 55.625) -> (87.9875, 54.625) centre (88.9875, 54.625) ccw
  line L168 (88.9875, 55.625) -> (90.0563, 55.625)
  line L169 (90.0563, 55.625) -> (90.0563, 58.675)
  arc A174 (91.0563, 59.675) -> (90.0563, 58.675) centre (91.0563, 58.675) ccw
  line L170 (91.0563, 59.675) -> (91.0563, 74.675)
  line L171 (91.0563, 74.675) -> (12.525, 74.675)
  arc A175 (12.525, 74.675) -> (11.05, 73.2) centre (12.525, 73.2) ccw
  line L172 (11.05, 73.2) -> (11.05, 58.15)
  arc A176 (8.525, 55.625) -> (11.05, 58.15) centre (8.525, 58.15) ccw
  line L173 (8.525, 55.625) -> (3, 55.625)
  arc A177 (3, 55.625) -> (1.525, 54.15) centre (3, 54.15) ccw
  line L174 (1.525, 54.15) -> (1.525, 3)
  arc A178 (1.525, 3) -> (3, 1.525) centre (3, 3) ccw
  line L175 (3, 1.525) -> (263.7, 1.525)
  arc A179 (263.7, 1.525) -> (265.175, 3) centre (263.7, 3) ccw
  line L176 (265.175, 3) -> (265.175, 54.15)
  arc A180 (265.175, 54.15) -> (263.7, 55.625) centre (263.7, 54.15) ccw
  line L177 (263.7, 55.625) -> (243.8875, 55.625)
  arc A181 (241.3625, 58.15) -> (243.8875, 55.625) centre (243.8875, 58.15) ccw
  line L178 (241.3625, 58.15) -> (241.3625, 73.2)
  arc A182 (241.3625, 73.2) -> (239.8875, 74.675) centre (239.8875, 73.2) ccw
  line L179 (239.8875, 74.675) -> (163.7375, 74.675)
  line L180 (163.7375, 74.675) -> (163.7375, 59.675)
  arc A183 (164.7375, 58.675) -> (163.7375, 59.675) centre (163.7375, 58.675) ccw
  line L181 (164.7375, 58.675) -> (164.7375, 55.625)
  line L182 (164.7375, 55.625) -> (168.1875, 55.625)
  arc A184 (169.1875, 54.625) -> (168.1875, 55.625) centre (168.1875, 54.625) ccw
  line L183 (169.1875, 54.625) -> (172.6875, 54.625)
  arc A185 (173.6875, 53.625) -> (172.6875, 54.625) centre (172.6875, 53.625) ccw
  line L184 (173.6875, 53.625) -> (173.6875, 41.625)
  arc A186 (172.6875, 40.625) -> (173.6875, 41.625) centre (172.6875, 41.625) ccw
  line L185 (172.6875, 40.625) -> (160.6875, 40.625)
  arc A187 (159.6875, 41.625) -> (160.6875, 40.625) centre (160.6875, 41.625) ccw
  line L186 (159.6875, 41.625) -> (159.6875, 53.625)
  arc A188 (159.6875, 53.625) -> (158.6875, 54.625) centre (158.6875, 53.625) ccw
  line L187 (158.6875, 54.625) -> (155.6375, 54.625)
  circle A189 centre (32.525, 66.675) radius 2
  circle A190 centre (47.625, 9.525) radius 2
  circle A191 centre (128.588, 37.025) radius 2
  circle A192 centre (220.025, 66.675) radius 2
  circle A193 centre (245.269, 9.525) radius 2
  dimension "d159" = 4
  dimension "d160" = 4
  dimension "d161" = 4
  dimension "d162" = 4
  dimension "d163" = 4
  constraint concentric A0 A189
  constraint concentric A9 A190
  constraint concentric A10 A191
  constraint concentric A36 A192
  constraint concentric A35 A193
  measures "d159" diameter of A189
  measures "d160" diameter of A190
  measures "d161" diameter of A191
  measures "d162" diameter of A192
  measures "d163" diameter of A193
extrude "Extrude9" add sketch "Sketch10" along normal blind 0.6 contours A189 | A190 | A191 | A192 | A193